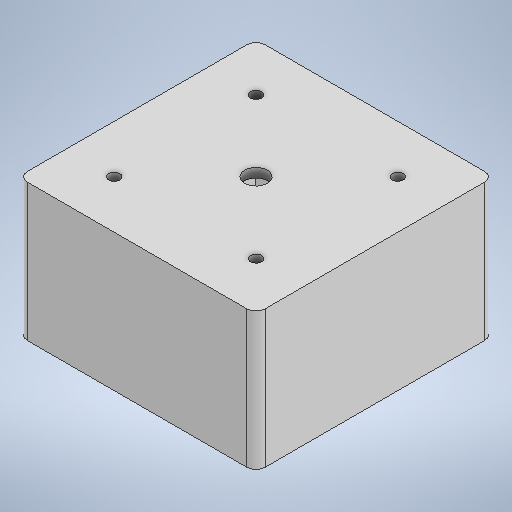
# Autodesk Inventor part: turnmotorcasing
Saved by Autodesk Inventor 2025.2 (Build 292293000, 293)
## iProperties
Created: 2026-03-22
Part Number: turnmotorcasing
Material: Generic
Document SubType Name: Modeling
Designer: hp
Density: 1 g/cm^3
Appearance: Default
Author: hp
Autodesk Inventor part; units mm, degrees
ref_plane "YZ Plane" through (0, 0, 0) normal (1, 0, 0) x (0, 1, 0)
ref_plane "XZ Plane" through (0, 0, 0) normal (0, 1, 0) x (-1, 0, 0)
ref_plane "XY Plane" through (0, 0, 0) normal (0, 0, 1) x (1, 0, 0)
sketch "Sketch1" plane through (0, 0, 0) normal (0, 1, 0) x (-1, 0, 0)
  line L0 (15.5, 15.5) -> (-15.5, 15.5)
  line L1 (-15.5, 15.5) -> (-15.5, -15.5)
  line L2 (-15.5, -15.5) -> (15.5, -15.5)
  line L3 (15.5, -15.5) -> (15.5, 15.5)
  line L4 (15.5, 15.5) -> (-15.5, -15.5) construction
  line L5 (-15.5, 15.5) -> (15.5, -15.5) construction
  line L6 (21, 21) -> (-21, 21)
  line L7 (-21, 21) -> (-21, -21)
  line L8 (-21, -21) -> (21, -21)
  line L9 (21, -21) -> (21, 21)
  line L10 (21, 21) -> (-21, -21) construction
  line L11 (-21, 21) -> (21, -21) construction
  line L12 (24, 26) -> (-24, 26)
  line L13 (-26, 24) -> (-26, -24)
  line L14 (-24, -26) -> (24, -26)
  line L15 (26, -24) -> (26, 24)
  circle A0 centre (0, 0) radius 2.5
  arc A1 (26, 24) -> (24, 26) centre (24, 24) ccw
  arc A2 (-24, 26) -> (-26, 24) centre (-24, 24) ccw
  arc A3 (24, -26) -> (26, -24) centre (24, -24) ccw
  arc A4 (-26, -24) -> (-24, -26) centre (-24, -24) ccw
  point P0 (26, 26)
  point P1 (-26, 26)
  point P2 (-26, -26)
  point P3 (26, -26)
  dimension "d0" = 31
  dimension "d1" = 31
  dimension "d2" = 42
  dimension "d3" = 42
  dimension "d4" = 5
  dimension "d7" = 5
  dimension "d23" = 2
  constraints: 32 end point, 8 point on circle, 8 point on line, 8 tangent, 6 parallel, 5 centre point, 4 midpoint, 3 equal radius, 3 perpendicular, 2 horizontal, 1 coincident, 3 other
  measures "d0" distance of L2.end L1.end
  measures "d1" distance of L1.end L0.end
  measures "d2" distance of L8.end L7.end
  measures "d3" distance of L7.end L6.end
  measures "d4" distance between parallel lines of L9 L15
  measures "d7" diameter of A0
  measures "d23" radius of A1
extrude "Extrusion1" add sketch "Sketch1" against normal blind 2 contours L3 L2 L1 L0 | L9 L8 L7 L6 | A0
extrude "Extrusion2" add sketch "Sketch1" against normal blind 30 contours A1 L15 A3 L14 A4 L13 A2 L12
hole "Hole1" at (-15.5, 0, -15.5) at (-15.5, 0, 15.5) at (15.5, 0, 15.5) at (15.5, 0, -15.5) direction (0, -1, 0) diameter 2.45 end through all
thread "Thread2" size "M2.5x0.45" class "6H" standard "ANSI Metric M Profile" full length
extrude "Extrusion3" cut sketch "Sketch1" against normal up to surface (2 mm away) contours A0
body "Solid1"
